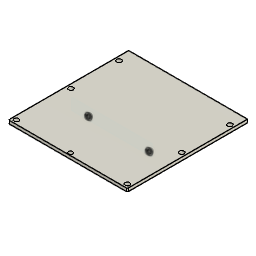
Mini Case - Rear Panel (Autodesk Fusion 360 design; units mm, degrees)
Autodesk Fusion 360 part; units mm, degrees
sketch "Sketch1" plane through (0, 0, 0) normal (0, 0, 1) x (1, 0, 0)
  line L0 (-56.8, 57.4) -> (56.8, 57.4)
  line L1 (56.8, 57.4) -> (56.8, -57.4)
  line L2 (56.8, -57.4) -> (-56.8, -57.4)
  line L3 (-56.8, -57.4) -> (-56.8, 57.4)
  point P0 (0, 57.4)
  point P1 (-56.8, 0)
  dimension "d1" = 113.6
  dimension "d2" = 114.8
  constraint horizontal L0
  constraint vertical L1
  constraint horizontal L2
  constraint vertical L3
  constraint midpoint L0 P0
  constraint midpoint L3 P1
  constraint vertical origin P0
  constraint horizontal origin P1
  measures "d1" distance of L0.start L0.end
  measures "d2" distance of L0.start L2.end
extrude "Extrude1" add sketch "Sketch1" along normal blind 3 makes body 1
sketch "Sketch2" plane through (0, 0, 3) normal (0, 0, 1) x (-1, 0, 0)
  line L0 (56.8, 57.4) -> (-56.8, 57.4)
  line L1 (-56.8, 57.4) -> (-56.8, -57.4)
  line L2 (-56.8, -57.4) -> (56.8, -57.4)
  line L3 (56.8, -57.4) -> (56.8, 57.4)
  circle A0 centre (53, -44.4) radius 2.25
  circle A1 centre (53, 1.6) radius 2.25
  circle A2 centre (53, 53.6) radius 2.25
  circle A3 centre (0.0159, 54.9) radius 2.05
  circle A4 centre (-53, 53.6) radius 2.25
  circle A5 centre (-53, 1.6) radius 2.25
  circle A6 centre (-53, -44.4) radius 2.25
  dimension "d5" = 4.5
  dimension "d6" = 4.5
  dimension "d7" = 4.5
  dimension "d9" = 4.5
  dimension "d10" = 4.5
  dimension "d11" = 4.5
  dimension "d12" = 3.8
  dimension "d13" = 3.8
  dimension "d14" = 2.5
  dimension "d16" = 13
  dimension "d17" = 46
  dimension "d18" = 52
  dimension "d19" = 4.1
  dimension "d20" = 53
  dimension "d21" = 53
  constraint vertical A0.centre A1.centre
  constraint vertical A1.centre A2.centre
  constraint vertical A4.centre A6.centre
  constraint vertical A5.centre A6.centre
  constraint horizontal A2.centre A4.centre
  constraint horizontal A1.centre A5.centre
  constraint horizontal A0.centre A6.centre
  measures "d5" diameter of A0
  measures "d6" diameter of A1
  measures "d7" diameter of A2
  measures "d9" diameter of A4
  measures "d10" diameter of A5
  measures "d11" diameter of A6
  measures "d12" distance of L3 A0.centre
  measures "d13" distance of L1 A6.centre
  measures "d14" distance of L0 A3.centre
  measures "d16" distance of L2 A0.centre
  measures "d17" distance of A0.centre A1.centre
  measures "d18" distance of A1.centre A2.centre
  measures "d19" diameter of A3
  measures "d20" distance of A2.centre A3.centre
extrude "Extrude2" cut sketch "Sketch2" against normal blind 3 contours A0 | A1 | A2 | A3 | A4 | A5 | A6 bodies 1
fillet "Fillet1" radius 1 2 edges at (-56.8, -57.4, 1.5) (56.8, -57.4, 1.5) on bodies 1
sketch "Sketch1 (1)" plane through (0, 0, 0) normal (0, 0, -1) x (1, 0, 0)
  arc A0 (56.8, 56.4) -> (55.8, 57.4) centre (55.8, 56.4) ccw
  line L0 (55.8, 57.4) -> (-55.8, 57.4)
  arc A1 (-55.8, 57.4) -> (-56.8, 56.4) centre (-55.8, 56.4) ccw
  line L1 (-56.8, 56.4) -> (-56.8, -57.4)
  line L2 (-56.8, -57.4) -> (56.8, -57.4)
  line L3 (56.8, -57.4) -> (56.8, 56.4)
  circle A2 centre (53, 53.6) radius 2.25
  circle A3 centre (-53, -44.4) radius 2.25
  circle A4 centre (-0.0159, 54.9) radius 2.05
  circle A5 centre (53, 1.6) radius 2.25
  circle A6 centre (-53, 1.6) radius 2.25
  circle A7 centre (-53, 53.6) radius 2.25
  circle A8 centre (53, -44.4) radius 2.25
  line L4 (28.6, 7.4) -> (-48.4, 7.4)
  line L5 (-48.4, 7.4) -> (-48.4, 5.4)
  line L6 (-48.4, 5.4) -> (28.6, 5.4)
  line L7 (28.6, 5.4) -> (28.6, 7.4)
  line L8 (-48.8, -51.4) -> (48.8, -51.4)
  line L9 (48.8, -51.4) -> (48.8, -54.4)
  line L10 (48.8, -54.4) -> (-48.8, -54.4)
  line L11 (-48.8, -54.4) -> (-48.8, -51.4)
  dimension "d26" = 77
  dimension "d27" = 2
  dimension "d39" = 8.4
  dimension "d45" = 52
  dimension "d46" = 8
  dimension "d47" = 8
  dimension "d50" = 3
  dimension "d51" = 3
  constraint horizontal L4
  constraint vertical L5
  constraint horizontal L6
  constraint vertical L7
  constraint horizontal L8
  constraint vertical L9
  constraint horizontal L10
  constraint vertical L11
  measures "d26" distance of L4.start L4.end
  measures "d27" distance of L4.start L6.end
  measures "d39" distance of L1 L5
  measures "d45" distance of L0 L6
  measures "d46" distance of L3 L9
  measures "d47" distance of L1 L11
  measures "d50" distance of L2 L10
  measures "d51" distance of L8 L10
extrude "Extrude4" add sketch "Sketch1 (1)" along normal blind 6 contours L8 L9 L10 L11 bodies 1
chamfer "Chamfer2" distance 6 angle 45 1 edges at (0, 51.4, 0) on bodies 1
extrude "Extrude1'" add sketch "Sketch1 (1)" along normal blind 11 contours L4 L5 L6 L7 bodies 1
chamfer "Chamfer1" distance 6 angle 45 1 edges at (-9.9, -7.4, 0) on bodies 1
sketch "Sketch2 (1)" plane through (0, -5.4, 0) normal (0, 1, 0) x (-1, 0, 0)
  line L0 (48.4, 0) -> (-28.6, 0)
  line L1 (-28.6, 0) -> (-28.6, -11)
  line L2 (-28.6, -11) -> (48.4, -11)
  line L3 (48.4, -11) -> (48.4, 0)
  circle A0 centre (32.4, -8) radius 1.425
  circle A1 centre (32.4, -8) radius 3
  circle A2 centre (-25.6, -8) radius 1.425
  circle A3 centre (-25.6, -8) radius 3
  dimension "d31" = 2.85
  dimension "d32" = 2.85
  dimension "d33" = 6
  dimension "d34" = 6
  dimension "d35" = 3
  dimension "d36" = 58
  dimension "d37" = 16
  constraint concentric A0 A1
  constraint concentric A2 A3
  constraint horizontal A0.centre A2.centre
  measures "d31" diameter of A0
  measures "d32" diameter of A2
  measures "d33" diameter of A1
  measures "d34" diameter of A3
  measures "d35" distance of L2 A0.centre
  measures "d36" horizontal distance of A0.centre A2.centre
  measures "d37" distance of L3 A0.centre
extrude "Extrude3" add sketch "Sketch2 (1)" along normal blind 5 separate body contours A1 | A3 makes body 2 at (22.6149, -2.0667, -7.7013) makes body 3 at (-35.3851, -2.0667, -7.7013)
extrude "Extrude2'" cut sketch "Sketch2 (1)" against normal blind 10 contours A0 | A2 bodies 1
sketch "Sketch3" plane through (0, 54.4, 0) normal (0, 1, 0) x (-1, 0, 0)
  line L0 (48.8, 0) -> (-48.8, 0)
  line L1 (-48.8, 0) -> (-48.8, -6)
  line L2 (-48.8, -6) -> (48.8, -6)
  line L3 (48.8, -6) -> (48.8, 0)
  line L4 (0, 0) -> (0, -6) construction
  circle A0 centre (0, -3) radius 1.425
  dimension "d55" = 2.85
  constraint coincident L4.start origin
  constraint midpoint L2 L4.end
  constraint midpoint L4 A0.centre
  measures "d55" diameter of A0
extrude "Extrude5" cut sketch "Sketch3" against normal blind 15 contours A0 bodies 1
equation "d6 = d5"
equation "d7 = d5"
equation "d9 = d5"
equation "d10 = d5"
equation "d11 = d5"
equation "d32 = d31"
equation "d34 = d33"
equation "d46 = d47"
named bodies: "Body1 (1)"
